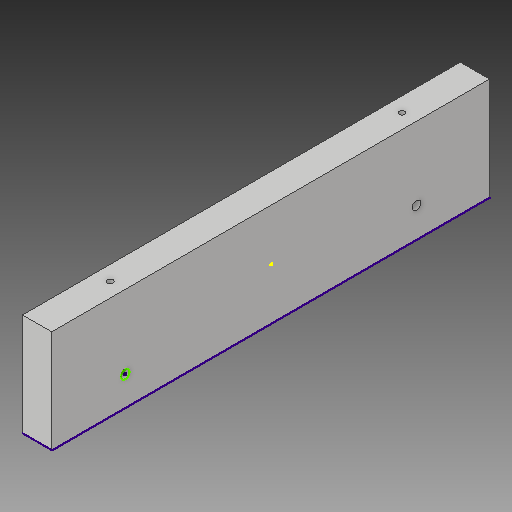
# Autodesk Inventor part: 马达安装版
Saved by Autodesk Inventor 2017 (Build 210142000, 142)
## iProperties
Part Number: 马达安装版
Material: 常规
Document SubType Name: Modeling
Designer: PANDA
Density: 1 g/cm^3
Appearance: 默认
Author: PANDA
Autodesk Inventor part; units mm, degrees
ref_plane "YZ Plane" through (0, 0, 0) normal (1, 0, 0) x (0, 1, 0)
ref_plane "XZ Plane" through (0, 0, 0) normal (0, 1, 0) x (-1, 0, 0)
ref_plane "XY Plane" through (0, 0, 0) normal (0, 0, 1) x (1, 0, 0)
sketch "草图1" plane through (0, 0, 0) normal (1, 0, 0) x (0, 1, 0)
  line L0 (35, 150) -> (-35, 150)
  line L1 (-35, 150) -> (-35, -150)
  line L2 (-35, -150) -> (35, -150)
  line L3 (35, -150) -> (35, 150)
  point P0 (0, 0)
  dimension "d0" = 70
  dimension "d1" = 300
  constraints: 8 end point, 2 parallel, 1 horizontal, 1 perpendicular
  measures "d0" distance of L2.end L1.end
  measures "d1" distance of L1.end L0.end
extrude "拉伸1" add sketch "草图1" along normal blind 20
sketch "草图2" plane through (0, 35, 150) normal (0, 1, 0) x (1, 0, 0)
  circle A0 centre (10, 50) radius 2
  point P0 (0, 150)
  dimension "d4" = 4
  constraints: 1 centre point
  measures "d4" diameter of A0
extrude "拉伸2" cut sketch "草图2" against normal blind 20
sketch "草图3" plane through (0, 35, 150) normal (0, 1, 0) x (1, 0, 0)
  circle A0 centre (10, 250) radius 2
  point P0 (0, 150)
  dimension "d7" = 4
  constraints: 1 centre point
  measures "d7" diameter of A0
extrude "拉伸3" cut sketch "草图3" against normal blind 40
sketch "草图4" plane through (20, 0, 0) normal (1, 0, 0) x (0, 0, -1)
  circle A0 centre (100, 0) radius 3
  point P0 (0, 0)
  dimension "d10" = 6
  constraints: 1 centre point
  measures "d10" diameter of A0
extrude "拉伸4" cut sketch "草图4" against normal through all
sketch "草图5" plane through (20, 0, 0) normal (1, 0, 0) x (0, 0, -1)
  circle A0 centre (-100, 0) radius 3
  point P0 (0, 0)
  dimension "d13" = 6
  constraints: 1 centre point
  measures "d13" diameter of A0
extrude "拉伸5" cut sketch "草图5" against normal through all
sketch "草图6" plane through (20, 0, 0) normal (1, 0, 0) x (0, 0, -1)
  circle A0 centre (-100, 0) radius 3 projected
  circle A1 centre (-100, 0) radius 3
  point P0 (0, 0)
  dimension "d16" = 6
  constraints: 1 centre point, 1 coincident
  measures "d16" diameter of A1
extrude "拉伸6" add sketch "草图6" against normal blind 20
sketch "草图7" plane through (20, 0, 0) normal (1, 0, 0) x (0, 0, -1)
  circle A0 centre (100, 0) radius 3 projected
  circle A1 centre (100, 0) radius 3
  point P0 (0, 0)
  dimension "d19" = 6
  constraints: 1 centre point, 1 coincident
  measures "d19" diameter of A1
extrude "拉伸7" add sketch "草图7" against normal blind 20
sketch "草图8" plane through (0, -35, -150) normal (0, -1, 0) x (1, 0, 0)
  line L0 (0, 300) -> (0, 0) projected
  line L1 (20, 300) -> (20, 0) projected
  line L2 (0, 300) -> (20, 300)
  line L3 (20, 300) -> (20, 0)
  line L4 (20, 0) -> (0, 0)
  line L5 (0, 0) -> (0, 300)
  point P0 (0, 150)
  constraints: 8 end point, 2 parallel, 1 horizontal, 1 perpendicular
sketch "草图9" plane through (20, 0, 0) normal (1, 0, 0) x (0, 0, -1)
  circle A0 centre (-100, -15) radius 3
  point P0 (0, 0)
  dimension "d22" = 6
  constraints: 1 centre point
  measures "d22" diameter of A0
extrude "拉伸8" cut sketch "草图9" against normal through all
sketch "草图10" plane through (20, 0, 0) normal (1, 0, 0) x (0, 0, -1)
  circle A0 centre (100, -15) radius 3
  point P0 (0, 0)
  dimension "d25" = 6
  constraints: 1 centre point
  measures "d25" diameter of A0
extrude "拉伸9" cut sketch "草图10" against normal through all
sketch "草图11" plane through (20, 0, 0) normal (1, 0, 0) x (0, 0, -1)
  circle A0 centre (-100, -15) radius 3 projected
  circle A1 centre (-100, -15) radius 3
  point P0 (0, 0)
  constraints: 1 centre point, 1 coincident
sketch "草图12" plane through (0, -35, -150) normal (0, -1, 0) x (1, 0, 0)
  point P0 (0, 150)
sketch "草图13" plane through (0, -35, -150) normal (0, -1, 0) x (1, 0, 0)
  point P0 (0, 150)
